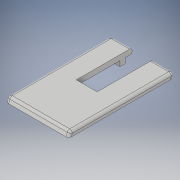
# Autodesk Inventor part: Lid
Saved by Autodesk Inventor 2019 (Build 230136000, 136)
## iProperties
Created: 2018-09-25
Part Number: Lid
Material: Generic
Document SubType Name: Modeling
Designer: mhall
Density: 1 g/cm^3
Appearance: Default
Author: mhall
Autodesk Inventor part; units mm, degrees
ref_plane "YZ Plane" through (0, 0, 0) normal (1, 0, 0) x (0, 1, 0)
ref_plane "XZ Plane" through (0, 0, 0) normal (0, 1, 0) x (-1, 0, 0)
ref_plane "XY Plane" through (0, 0, 0) normal (0, 0, 1) x (1, 0, 0)
sketch "Sketch1" plane through (0, 0, 0) normal (0, 1, 0) x (-1, 0, 0)
  line L0 (0, 0) -> (60.96, 0)
  line L1 (60.96, 0) -> (60.96, -111.76)
  line L2 (60.96, -111.76) -> (0, -111.76)
  line L3 (0, -111.76) -> (0, 0)
  dimension "d0" = 60.96
  dimension "d1" = 111.76
  constraints: 8 end point, 2 parallel, 1 horizontal, 1 perpendicular
  measures "d0" distance of L1.end L2.end
  measures "d1" distance of L0.end L1.end
extrude "Extrusion1" add sketch "Sketch1" along normal blind 6.35
sketch "Sketch2" plane through (0, 6.35, 0) normal (0, 1, 0) x (1, 0, 0)
  line L0 (-60.96, 0) -> (0, 0) projected
  line L1 (0, 0) -> (0, 111.76) projected
  line L2 (0, 111.76) -> (-60.96, 111.76) projected
  line L3 (-60.96, 111.76) -> (-60.96, 0) projected
  line L4 (7.62, -7.62) -> (-68.58, -7.62)
  line L5 (-68.58, -7.62) -> (-68.58, 119.38)
  line L6 (-68.58, 119.38) -> (7.62, 119.38)
  line L7 (7.62, 119.38) -> (7.62, -7.62)
  dimension "d4" = 7.62
  constraints: 8 end point, 3 other
  measures "d4" distance between parallel lines of L0 L4
extrude "Extrusion2" add sketch "Sketch2" along normal blind 6.35 contours L3 L2 L1 L0 | L4 L5 L6 L7
sketch "Sketch3" plane through (7.62, 6.35, 7.62) normal (1, 0, 0) x (0, 0, -1)
  line L0 (127, 0) -> (127, 6.35) projected
  line L1 (127, 0) -> (129.0632, 6.35)
  line L2 (127, 0) -> (136.5189, 0) construction
  line L3 (127, 6.35) -> (129.0632, 6.35)
  line L4 (0, 0) -> (0, 6.35) projected
  line L5 (0, 0) -> (2.0632, 6.35)
  line L6 (127, 6.35) -> (0, 6.35) projected
  line L7 (127, 0) -> (0, 0) projected
  line L8 (127, 0) -> (127, 6.35) projected
  line L9 (0, 6.35) -> (127, 6.35) projected
  line L10 (0, 0) -> (0, 6.35) projected
  point P0 (7.62, -6.35)
  dimension "d7" = 72
  constraints: 8 end point, 2 horizontal, 1 point on line
  measures "d7" angle of L2 L1
extrude "Extrusion3" add sketch "Sketch3" against normal blind 76.2 contours L0 L3 L1 | L4 L6 L5
sketch "Sketch4" plane through (7.62, 6.35, 7.62) normal (1, 0, 0) x (0, 0, -1)
  line L0 (0, 0) -> (2.0632, 6.35)
  line L1 (0, 0) -> (11.0448, 0) construction
  line L2 (0, 0) -> (0, 6.35) projected
  line L3 (0, 6.35) -> (129.0632, 6.35) projected
  point P0 (7.62, -6.35)
  dimension "d10" = 72
  constraints: 4 end point, 1 horizontal, 1 point on line
  measures "d10" angle of L1 L0
extrude "Extrusion4" cut sketch "Sketch4" against normal through all
fillet "Fillet2" radius 3.175 8 edges at (-68.58, 12.7, -57.9432) (-30.48, 12.7, -121.4432) (7.62, 12.7, -57.9432) (-68.58, 9.525, -120.4116) (7.62, 9.525, -120.4116) (7.62, 9.525, 6.5884) (-68.58, 9.525, 6.5884) (-30.48, 12.7, 5.5568)
sketch "Sketch5" plane through (0, 0, 0) normal (0, -1, 0) x (1, 0, 0)
  line L0 (0, 0) -> (-60.96, 0) projected
  line L1 (-60.96, 0) -> (-60.96, -111.76) projected
  line L2 (-60.96, -111.76) -> (0, -111.76) projected
  line L3 (0, -111.76) -> (0, 0) projected
  line L4 (-6.35, -6.35) -> (-54.61, -6.35)
  line L5 (-54.61, -6.35) -> (-54.61, -105.41)
  line L6 (-54.61, -105.41) -> (-6.35, -105.41)
  line L7 (-6.35, -105.41) -> (-6.35, -6.35)
  dimension "d16" = 6.35
  constraints: 8 end point, 3 other
  measures "d16" distance between parallel lines of L3 L7
extrude "Extrusion5" cut sketch "Sketch5" against normal blind 6.35 contours L7 L6 L5 L4
sketch "Sketch6" plane through (0, 0, 0) normal (0, -1, 0) x (1, 0, 0)
  line L0 (-60.96, -111.76) -> (0, -111.76) projected
  line L1 (-30.48, -111.76) -> (-17.78, -111.76)
  line L2 (-6.35, -105.41) -> (-54.61, -105.41) projected
  line L3 (-17.78, -111.76) -> (-43.18, -111.76)
  line L4 (-43.18, -111.76) -> (-43.18, -105.41)
  line L5 (-43.18, -105.41) -> (-17.78, -105.41)
  line L6 (-17.78, -105.41) -> (-17.78, -111.76)
  point P0 (0, 0)
  dimension "d19" = 12.7
  dimension "d20" = 25.4
  constraints: 10 end point, 2 parallel, 2 point on line, 1 horizontal, 1 midpoint, 1 perpendicular
  measures "d19" distance of L1.start L1.end
  measures "d20" distance of L4.end L5.end
extrude "Extrusion6" cut sketch "Sketch6" against normal blind 6.35
sketch "Sketch7" plane through (0, 6.35, 0) normal (0, -1, 0) x (1, 0, 0)
  line L0 (-17.78, -105.41) -> (-17.78, -111.76) projected
  line L1 (-17.78, -111.76) -> (-43.18, -111.76)
  line L2 (-43.18, -111.76) -> (-43.18, -142.1145)
  line L3 (-43.18, -142.1145) -> (-17.78, -142.1145)
  line L4 (-17.78, -142.1145) -> (-17.78, -111.76)
  line L5 (-43.18, -142.1145) -> (-17.78, -142.1145)
  line L6 (-17.78, -142.1145) -> (-17.78, -89.8971)
  line L7 (-17.78, -89.8971) -> (-43.18, -89.8971)
  line L8 (-43.18, -89.8971) -> (-43.18, -142.1145)
  point P0 (0, 0)
  constraints: 16 end point, 4 parallel, 2 horizontal, 2 perpendicular, 1 point on line
extrude "Extrusion7" cut sketch "Sketch7" against normal blind 25.4
sketch "Sketch8" plane through (0, 6.35, 0) normal (0, -1, 0) x (1, 0, 0)
  line L0 (-43.18, -89.8971) -> (-17.78, -89.8971) projected
  line L1 (-17.78, -89.8971) -> (-43.18, -89.8971)
  line L2 (-43.18, -89.8971) -> (-43.18, -52.3331)
  line L3 (-43.18, -52.3331) -> (-17.78, -52.3331)
  line L4 (-17.78, -52.3331) -> (-17.78, -89.8971)
  point P0 (0, 0)
  constraints: 8 end point, 2 parallel, 1 horizontal, 1 perpendicular
extrude "Extrusion8" cut sketch "Sketch8" against normal blind 25.4
body "Solid1"
